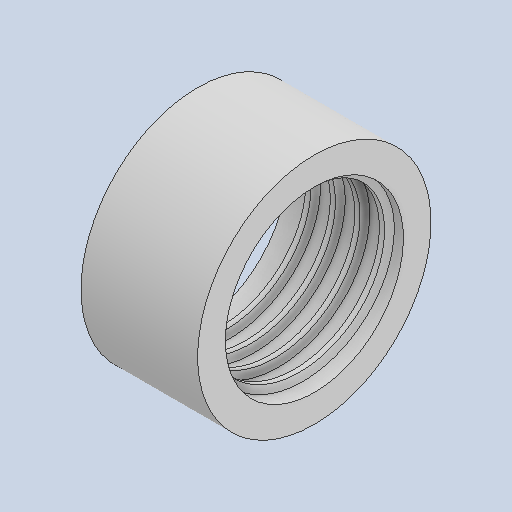
# Autodesk Inventor part: secrure_ring
Saved by Autodesk Inventor 2025 (Build 290162000, 162)
## iProperties
Created: 2026-04-08
Part Number: secrure_ring
Material: Generic
Document SubType Name: Modeling
Designer: Luca
Density: 1 g/cm^3
Appearance: Default
Author: Luca
Autodesk Inventor part; units mm, degrees
ref_plane "YZ Plane" through (0, 0, 0) normal (1, 0, 0) x (0, 1, 0)
ref_plane "XZ Plane" through (0, 0, 0) normal (0, 1, 0) x (-1, 0, 0)
ref_plane "XY Plane" through (0, 0, 0) normal (0, 0, 1) x (1, 0, 0)
derived "sk_reservoir.ipt"
sketch "pipe_out" plane through (-77.5, 0, 0) normal (1, 0, 0) x (0, 1, 0)
  line L0 (-132, 0) -> (302, 0)
  circle A0 centre (-10, 0) radius 7.5
  line L1 (0, 153.4424) -> (0, -148.4939)
  circle A1 centre (-10, 0) radius 7.25
  circle A2 centre (-10, 0) radius 5
  circle A3 centre (-10, 0) radius 9.5
  circle A4 centre (-10, 0) radius 6
  circle A5 centre (-10, 0) radius 6.25
  circle A6 centre (-10, 0) radius 9.75
  point P0 (0, 0)
  point P1 (-2.5, 0)
  point P2 (-2.75, 0)
ref_plane "Work Plane1" through (0, 240, 0) normal (0, 1, 0) x (-1, 0, 0)
ref_plane "bottom_plane" through (0, -70, 0) normal (0, 1, 0) x (-1, 0, 0)
ref_plane "water_bottom" through (0, -67, 0) normal (0, 1, 0) x (-1, 0, 0)
ref_plane "mount_top" through (0, -66, 0) normal (0, 1, 0) x (-1, 0, 0)
ref_plane "hull_hole_top" through (0, -65.9, 0) normal (0, 1, 0) x (-1, 0, 0)
ref_plane "hull_mount_top" through (0, -57.9, 0) normal (0, 1, 0) x (-1, 0, 0)
ref_plane "motor_mount_plane" through (0, -54, 0) normal (0, 1, 0) x (-1, 0, 0)
ref_plane "button_back" through (-77.5, 0, 0) normal (1, 0, 0) x (0, 1, 0)
ref_plane "battery_lid_top" through (0, -1, 0) normal (0, 1, 0) x (-1, 0, 0)
ref_plane "lid_magnet_center" through (0, 2, 0) normal (0, 1, 0) x (-1, 0, 0)
ref_plane "lid_upper_top" through (0, 4, 0) normal (0, 1, 0) x (-1, 0, 0)
ref_plane "lid_lower_top" through (0, 1.9, 0) normal (0, 1, 0) x (-1, 0, 0)
ref_plane "lid_upper_bottom" through (0, 2, 0) normal (0, 1, 0) x (-1, 0, 0)
extrude "Extrusion1" add sketch "pipe_out" along normal blind 9.5 contours A1 L0 A0 | L0 A0 A1 | A0 L0 A3 | L0 A3 A0
sketch "Sketch22" plane through (0, 0, 0) normal (0, 0, 1) x (1, 0, 0)
  line L0 (-77.5, -10) -> (-82.5, -10) projected
  arc A0 (-102.5, 10) -> (-82.5, -10) centre (-82.5, 10) ccw projected
  line L1 (-77.5, -10) -> (-67.5, -10) projected
  line L2 (-77.5, -2.75) -> (-76, -2.75) projected
  line L3 (-76.433, -3.5) -> (-77.067, -3.5) projected
  line L4 (-76.25, -2.75) -> (-76.5387, -3.25) projected
  line L5 (-76.5387, -3.25) -> (-76.9613, -3.25) projected
  line L6 (-76.9613, -3.25) -> (-77.25, -2.75) projected
  line L7 (-76.75, -2.75) -> (-76.75, -3.5) construction
  line L8 (-76, -2.75) -> (-76.433, -3.5) projected
  line L9 (-77.5, -2.75) -> (-77.067, -3.5) projected
  point P0 (0, 0)
  point P1 (-77.5, -2.5)
coil "Coil1" sketch "Sketch22" operation add axis through (-77.5, -10, 0) along (1, 0, 0) pitch 2 turns 4 hand right contours L2 L4 L5 L6
ref_plane "Work Plane23" through (0, 0, 72) normal (0, 0, 1) x (1, 0, 0)
ref_plane "Work Plane26" through (0, -3, 0) normal (0, 1, 0) x (-1, 0, 0)
ref_plane "Work Plane32" through (-82.5, -10, 0) normal (-1, 0, 0) x (0, -1, 0)
body "Solid1"
